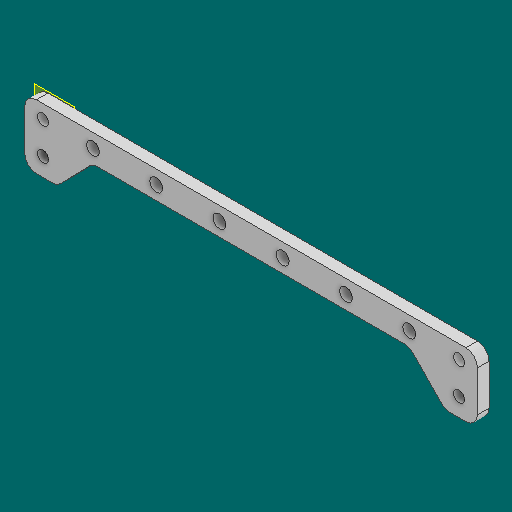
# Autodesk Inventor part: string_mount
Saved by Autodesk Inventor 2023 (Build 270158000, 158)
## iProperties
Created: 2022-11-12
Part Number: string_mount
Material: Generic
Document SubType Name: Modeling
Designer: sgodi
Density: 1 g/cm^3
Appearance: Default
Author: sgodi
Autodesk Inventor part; units mm, degrees
ref_plane "YZ Plane" through (0, 0, 0) normal (1, 0, 0) x (0, 1, 0)
ref_plane "XZ Plane" through (0, 0, 0) normal (0, 1, 0) x (-1, 0, 0)
ref_plane "XY Plane" through (0, 0, 0) normal (0, 0, 1) x (1, 0, 0)
ref_plane "Work Plane2" through (0, 147.11, 157.65) normal (0, 0, 1) x (1, 0, 0)
sketch "Sketch2" plane through (0, 147.11, 157.65) normal (0, 0, 1) x (1, 0, 0)
  arc A0 (61.9417, -3.175) -> (58.7667, 0) centre (58.7667, -3.175) ccw projected
  line L0 (58.7667, 0) -> (55.1167, 0) projected
  arc A1 (51.9417, 3.175) -> (55.1167, 0) centre (55.1167, 3.175) ccw projected
  arc A2 (51.9417, 3.937) -> (48.7667, 7.112) centre (48.7667, 3.937) ccw projected
  line L1 (48.7667, 7.112) -> (-48.7667, 7.112) projected
  arc A3 (-48.7667, 7.112) -> (-51.9417, 3.937) centre (-48.7667, 3.937) ccw projected
  arc A4 (-55.1167, 0) -> (-51.9417, 3.175) centre (-55.1167, 3.175) ccw projected
  line L2 (-55.1167, 0) -> (-58.7667, 0) projected
  arc A5 (-58.7667, 0) -> (-61.9417, -3.175) centre (-58.7667, -3.175) ccw projected
  line L3 (-61.9417, -3.175) -> (-61.9417, -14.325) projected
  arc A6 (-61.9417, -14.325) -> (-58.7667, -17.5) centre (-58.7667, -14.325) ccw projected
  line L4 (-58.7667, -17.5) -> (-54.3979, -17.5) projected
  arc A7 (-54.3979, -17.5) -> (-52.1213, -16.5381) centre (-54.3979, -14.325) ccw projected
  line L5 (-52.1213, -16.5381) -> (-44.2704, -8.4619) projected
  arc A8 (-41.9938, -7.5) -> (-44.2704, -8.4619) centre (-41.9938, -10.675) ccw projected
  line L6 (-41.9938, -7.5) -> (41.9938, -7.5) projected
  arc A9 (44.2704, -8.4619) -> (41.9938, -7.5) centre (41.9938, -10.675) ccw projected
  line L7 (44.2704, -8.4619) -> (52.1213, -16.5381) projected
  arc A10 (52.1213, -16.5381) -> (54.3979, -17.5) centre (54.3979, -14.325) ccw projected
  line L8 (54.3979, -17.5) -> (58.7667, -17.5) projected
  arc A11 (58.7667, -17.5) -> (61.9417, -14.325) centre (58.7667, -14.325) ccw projected
  line L9 (61.9417, -14.325) -> (61.9417, -3.175) projected
  arc A12 (-44.4178, 0) -> (-42.1518, 0) centre (-43.2848, 0) ccw projected
  line L10 (-44.4178, 0) -> (-44.4178, 5) projected
  arc A13 (-42.1518, 5) -> (-44.4178, 5) centre (-43.2848, 5) ccw projected
  line L11 (-42.1518, 5) -> (-42.1518, 0) projected
  circle A14 centre (56.9417, -12.5) radius 1.524 projected
  circle A15 centre (-56.9417, -3.75) radius 1.524 projected
  circle A16 centre (56.9417, -3.75) radius 1.524 projected
  circle A17 centre (-43.2848, -3.75) radius 1.27 projected
  circle A18 centre (-25.9709, -3.75) radius 1.27 projected
  circle A19 centre (-8.657, -3.75) radius 1.27 projected
  circle A20 centre (8.657, -3.75) radius 1.27 projected
  circle A21 centre (25.9709, -3.75) radius 1.27 projected
  circle A22 centre (43.2848, -3.75) radius 1.27 projected
  circle A23 centre (-56.9417, -12.5) radius 1.524 projected
  arc A24 (-27.1039, 0) -> (-24.8379, 0) centre (-25.9709, 0) ccw projected
  line L12 (-27.1039, 0) -> (-27.1039, 5) projected
  arc A25 (-24.8379, 5) -> (-27.1039, 5) centre (-25.9709, 5) ccw projected
  line L13 (-24.8379, 5) -> (-24.8379, 0) projected
  arc A26 (-9.79, 0) -> (-7.524, 0) centre (-8.657, 0) ccw projected
  line L14 (-9.79, 0) -> (-9.79, 5) projected
  arc A27 (-7.524, 5) -> (-9.79, 5) centre (-8.657, 5) ccw projected
  line L15 (-7.524, 5) -> (-7.524, 0) projected
  arc A28 (7.524, 0) -> (9.79, 0) centre (8.657, 0) ccw projected
  line L16 (7.524, 0) -> (7.524, 5) projected
  arc A29 (9.79, 5) -> (7.524, 5) centre (8.657, 5) ccw projected
  line L17 (9.79, 5) -> (9.79, 0) projected
  arc A30 (24.8379, 0) -> (27.1039, 0) centre (25.9709, 0) ccw projected
  line L18 (24.8379, 0) -> (24.8379, 5) projected
  arc A31 (27.1039, 5) -> (24.8379, 5) centre (25.9709, 5) ccw projected
  line L19 (27.1039, 5) -> (27.1039, 0) projected
  arc A32 (42.1518, 0) -> (44.4178, 0) centre (43.2848, 0) ccw projected
  line L20 (42.1518, 0) -> (42.1518, 5) projected
  arc A33 (44.4178, 5) -> (42.1518, 5) centre (43.2848, 5) ccw projected
  line L21 (44.4178, 5) -> (44.4178, 0) projected
  line L22 (-55.1167, 0) -> (55.1167, 0)
  circle A34 centre (-43.2848, -3.75) radius 1.778
  circle A35 centre (-25.9709, -3.75) radius 1.778
  circle A36 centre (-8.657, -3.75) radius 1.778
  circle A37 centre (8.657, -3.75) radius 1.778
  circle A38 centre (25.9709, -3.75) radius 1.778
  circle A39 centre (43.2848, -3.75) radius 1.778
  line L23 (51.9417, 3.175) -> (51.9417, 3.937) projected
  line L24 (-51.9417, 3.937) -> (-51.9417, 3.175) projected
  point P0 (0, -147.11)
  point P1 (51.9417, 3.683)
  point P2 (-51.9417, 3.683)
  dimension "d0" = 3.556
  dimension "d1" = 3.556
  dimension "d2" = 3.556
  dimension "d3" = 3.556
  dimension "d4" = 3.556
  dimension "d5" = 3.556
  constraints: 6 centre point, 6 coincident, 2 end point, 1 collinear, 1 tangent
  measures "d0" diameter of A34
  measures "d1" diameter of A35
  measures "d2" diameter of A36
  measures "d3" diameter of A37
  measures "d4" diameter of A38
  measures "d5" diameter of A39
extrude "Extrusion1" add sketch "Sketch2" along normal blind 3.175 contours L9 A11 L8 A10 L7 A9 L6 A8 L5 A7 L4 A6 L3 A5 L2 L22 A12 A24 A26 A28 A30 A32 L0 A0 | A32 L22 | A30 L22 | A28 L22 | A26 L22 | L22 A12 | A24 L22
body "Solid1"
